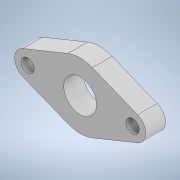
# Autodesk Inventor part: 1.6
Saved by Autodesk Inventor 2022 (Build 260153000, 153)
## iProperties
Created: 2023-04-17
Part Number: 1.6
Material: Genérico
Document SubType Name: Modeling
Designer: jpjoa
Density: 1 g/cm^3
Appearance: Padrão
Author: jpjoa
Autodesk Inventor part; units mm, degrees
ref_plane "YZ Plane" through (0, 0, 0) normal (1, 0, 0) x (0, 1, 0)
ref_plane "XZ Plane" through (0, 0, 0) normal (0, 1, 0) x (-1, 0, 0)
ref_plane "XY Plane" through (0, 0, 0) normal (0, 0, 1) x (1, 0, 0)
sketch "Esboço1" plane through (0, 0, 0) normal (0, 0, 1) x (1, 0, 0)
  circle A0 centre (0, 0) radius 12.5
  circle A1 centre (-40, 0) radius 5
  circle A2 centre (40, 0) radius 5
  circle A3 centre (-40, 0) radius 10
  circle A4 centre (40, 0) radius 10
  circle A5 centre (0, 0) radius 25
  line L0 (-43.75, 9.2702) -> (-9.375, 23.1756)
  line L1 (-43.75, -9.2702) -> (-9.375, -23.1756)
  line L2 (43.75, -9.2702) -> (9.375, -23.1756)
  line L3 (9.375, 23.1756) -> (43.75, 9.2702)
  dimension "d0" = 25
  dimension "d1" = 10
  dimension "d2" = 10
  dimension "d3" = 40
  dimension "d4" = 80
  dimension "d5" = 20
  dimension "d6" = 20
  dimension "d7" = 50
  constraints: 8 end point, 8 point on circle, 8 tangent, 6 centre point, 3 concentric, 2 horizontal alignment, 1 coincident
  measures "d0" diameter of A0
  measures "d1" diameter of A1
  measures "d2" diameter of A2
  measures "d3" distance of A2.centre point (0, 0)
  measures "d4" distance of A2.centre A1.centre
  measures "d5" diameter of A3
  measures "d6" diameter of A4
  measures "d7" diameter of A5
extrude "Extrusão1" add sketch "Esboço1" along normal blind 15
